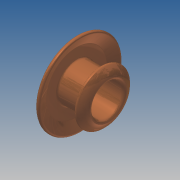
# Autodesk Inventor part: wstawka
Saved by Autodesk Inventor 2012 SP1 (Build 160190100, 190)
## iProperties
Created: 2012-12-05
Part Number: wstawka
Material: Miedziany
Document SubType Name: Modeling
Designer: Komp
Density: 8.94 g/cm^3
Mass: 0.0999458 g
Surface Area: 1.02317 cm^2
Volume: 0.0111796 cm^3
Author: Komp
Autodesk Inventor part; units mm, degrees
ref_plane "YZ Plane" through (0, 0, 0) normal (1, 0, 0) x (0, 1, 0)
sketch "Szkic1" plane through (0, 0, 0) normal (0, 0, 1) x (1, 0, 0)
  line L0 (0, 1.25) -> (1, 1.25)
  line L1 (0, 0) -> (4.8685, 0)
  line L2 (0.625, 1.8) -> (0.8471, 1.5669)
  line L3 (0.8471, 1.5669) -> (1, 1.25)
  line L4 (0, 1.25) -> (-1, 1.25)
  line L5 (-1, 1.25) -> (-0.9671, 2.0325)
  line L6 (-0.9671, 2.0325) -> (-0.625, 2.8)
  line L7 (1.2, 1.25) -> (1.2, 1.05)
  line L8 (1.2, 1.05) -> (-1.2441, 1.05)
  line L9 (-0.8691, 2.8) -> (-0.625, 2.8)
  line L10 (0.625, 1.8) -> (0.825, 1.8)
  arc A0 (-0.8691, 2.8) -> (-1.2441, 1.05) centre (1.098, 1.4633) ccw
  arc A1 (1.2, 1.25) -> (0.825, 1.8) centre (0.1585, 0.9427) ccw
  line L11 (1.2, 1.25) -> (1.2, 1.05)
  dimension "d1" = 1
  dimension "d16" = 0.2
  constraints: 24 end point, 4 point on circle, 2 centre point, 2 parallel, 2 perpendicular
  measures "d1" distance of L0.start L0.end
  measures "d16" distance of L11.start L11.end
revolve "Obrót1" add sketch "Szkic1" angle 360 about axis through (0, 0, 0) along (1, 0, 0)
fillet "Zaokrąglenie1" radius 0.2 2 edges at (-1.2441, -1.05, 0) (1.2, -1.05, 0)
fillet "Zaokrąglenie2" radius 0.1 7 edges at (0.825, -1.8, 0) (1, -1.25, 0) (0.8471, -1.5669, 0) (-0.8691, -2.8, 0) (-0.625, -2.8, 0) (-0.9671, -2.0325, 0) (-1, -1.25, 0)
fillet "Zaokrąglenie3" radius 0.05 1 edges at (0.625, -1.8, 0)
ref_plane "Płaszczyzna konstrukcyjna1" through (0, 0, 0) normal (0, 1, 0) x (-1, 0, 0)
ref_plane "Płaszczyzna konstrukcyjna2" through (0, 0, 0) normal (0, 0, 1) x (1, 0, 0)
